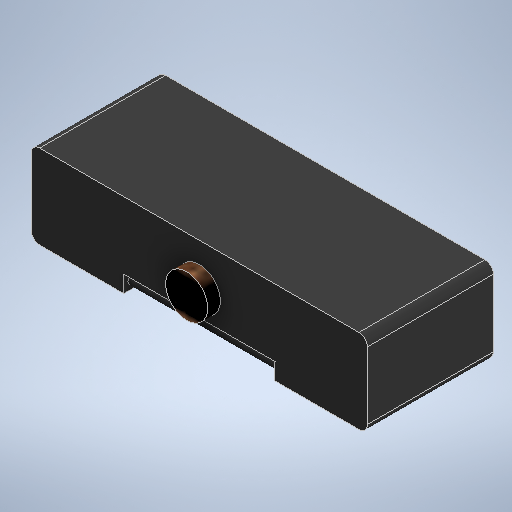
# Autodesk Inventor part: Caja
Saved by Autodesk Inventor 2025.2 (Build 292293000, 293)
## iProperties
Created: 2025-06-29
Part Number: Caja
Material: Rubber, Silicone
Document SubType Name: Sheet Metal
Designer: asus
Mass: 7.5 g
Surface Area: 23 cm^2
Volume: 6 cm^3
Density: 1.25 g/cm^3
Sheet Metal Rule: Default
Appearance: Rubber - Black
Author: asus
Autodesk Inventor part; units mm, degrees
ref_plane "YZ Plane" through (0, 0, 0) normal (1, 0, 0) x (0, 1, 0)
ref_plane "XZ Plane" through (0, 0, 0) normal (0, 1, 0) x (-1, 0, 0)
ref_plane "XY Plane" through (0, 0, 0) normal (0, 0, 1) x (1, 0, 0)
sketch "Sketch1" plane through (0, 0, 0) normal (0, 0, 1) x (1, 0, 0)
  line L0 (0, 1) -> (0, 9)
  line L1 (1, 10) -> (39, 10)
  line L2 (40, 9) -> (40, 1)
  line L3 (39, 0) -> (1, 0)
  arc A0 (1, 10) -> (0, 9) centre (1, 9) ccw
  arc A1 (40, 9) -> (39, 10) centre (39, 9) ccw
  arc A2 (39, 0) -> (40, 1) centre (39, 1) ccw
  arc A3 (0, 1) -> (1, 0) centre (1, 1) ccw
  point P0 (0, 0)
  point P1 (0, 10)
  point P2 (40, 10)
  point P3 (40, 0)
  dimension "d0" = 10
  dimension "d1" = 40
  dimension "d4" = 1
  constraints: 8 end point, 8 point on circle, 8 point on line, 8 tangent, 4 centre point, 3 equal radius, 2 perpendicular, 1 horizontal, 1 vertical
  measures "d0" distance of point (0, 0) point (0, 10)
  measures "d1" distance of point (0, 10) point (40, 10)
  measures "d4" radius of A0
extrude "Extrusion1" add sketch "Sketch1" against normal blind 15
sketch "Sketch2" plane through (1, 0, 0) normal (0, -1, 0) x (1, 0, 0)
  line L0 (0, 0) -> (38, 0) projected
  line L1 (0, 0) -> (0, -15) projected
  line L2 (38, -15) -> (0, -15) projected
  line L3 (38, 0) -> (38, -15) projected
  line L4 (0, 0) -> (38, 0) projected
  line L5 (0, 0) -> (0, -15) projected
  line L6 (38, -15) -> (0, -15) projected
  line L7 (38, 0) -> (38, -15) projected
  line L8 (0, 0) -> (38, 0) projected
  line L9 (38, -15) -> (0, -15) projected
  line L10 (0, 0) -> (0, -15) projected
  line L11 (38, 0) -> (38, -15) projected
  line L12 (16.2, -5.85) -> (16.2, -9.15)
  line L13 (16.2, -9.15) -> (21.8, -9.15)
  line L14 (21.8, -9.15) -> (21.8, -5.85)
  line L15 (21.8, -5.85) -> (16.2, -5.85)
  point P0 (-1, 0)
  point P1 (16.2, -7.5)
  dimension "d8" = 3.3
  dimension "d9" = 5.6
  dimension "d10" = 16.2
  dimension "d11" = 5.85
  constraints: 8 end point, 3 perpendicular, 1 midpoint, 1 vertical
  measures "d8" distance of L12.start L12.end
  measures "d9" distance of L12.end L13.end
  measures "d10" distance from line of point (16.2, -7.5) L1
  measures "d11" distance between parallel lines of L0 L15
extrude "Extrusion2" cut sketch "Sketch2" against normal blind 1.6 contours L15 L14 L13 L12
sketch "Sketch3" plane through (0, 0, 0) normal (0, 0, 1) x (1, 0, 0)
  line L0 (40, 1) -> (40, 9) projected
  arc A0 (40, 9) -> (39, 10) centre (39, 9) ccw projected
  line L1 (39, 10) -> (1, 10) projected
  arc A1 (1, 10) -> (0, 9) centre (1, 9) ccw projected
  line L2 (0, 9) -> (0, 1) projected
  arc A2 (0, 1) -> (1, 0) centre (1, 1) ccw projected
  line L3 (1, 0) -> (39, 0) projected
  arc A3 (39, 0) -> (40, 1) centre (39, 1) ccw projected
  circle A4 centre (20, 5) radius 2.5
  point P0 (0, 0)
  dimension "d14" = 5
  constraints: 1 centre point
  measures "d14" diameter of A4
extrude "Extrusion3" add sketch "Sketch3" along normal blind 1.5 contours A4
sketch "Sketch4" plane through (0, 0, 0) normal (0, 0, 1) x (1, 0, 0)
  line L0 (17.2, 0) -> (22.8, 0) projected
  line L1 (20, 0) -> (11, 0)
  line L2 (1, 0) -> (39, 0) projected
  line L3 (11, 0) -> (11, 2)
  line L4 (11, 2) -> (29, 2)
  line L5 (29, 2) -> (29, 0)
  line L6 (29, 0) -> (20, 0)
  point P0 (0, 0)
  point P1 (29, 0)
  dimension "d17" = 9
  dimension "d18" = 2
  dimension "d19" = 18
  constraints: 10 end point, 3 perpendicular, 2 point on line, 1 collinear, 1 midpoint
  measures "d17" distance of L1.start L1.end
  measures "d18" distance of L1.end L3.end
  measures "d19" distance of L3.end L4.end
extrude "Extrusion4" cut sketch "Sketch4" against normal blind 2
sketch "Sketch5" plane through (0, 0, -15) normal (0, 0, -1) x (-1, 0, 0)
  line L0 (-11, 2) -> (-29, 2) projected
  line L1 (-11, 0) -> (-11, 2) projected
  line L2 (-39, 0) -> (-1, 0) projected
  line L3 (-29, 2) -> (-29, 0) projected
  point P0 (0, 0)
extrude "Extrusion5" cut sketch "Sketch5" against normal blind 2
sketch "Sketch6" plane through (11, 0, 0) normal (1, 0, 0) x (0, 0, -1)
  circle A0 centre (1.0103, 0.9523) radius 0.5
  point P0 (0, 0)
  dimension "d24" = 1
  constraints: 1 centre point
  measures "d24" diameter of A0
extrude "Extrusion6" add sketch "Sketch6" along normal blind 18
sketch "Sketch7" plane through (11, 0, -15) normal (1, 0, 0) x (0, 0, -1)
  circle A0 centre (-0.8887, 1) radius 0.5
  point P0 (-15, 0)
  dimension "d27" = 1
  constraints: 1 centre point
  measures "d27" diameter of A0
extrude "Extrusion7" add sketch "Sketch7" along normal blind 18
equation "\"BendRadius\" = Thickness"
equation "\"BendReliefWidth\" = Thickness"
equation "\"BendReliefDepth\" = 0.5 * Thickness"
equation "\"CornerReliefSize\" = 4 * Thickness"
equation "\"MinimumRemnant\" = 2 * Thickness"
equation "\"TransitionRadius\" = BendRadius"
equation "\"JacobiRadiusSize\" = BendRadius"
equation "\"GapSize\" = Thickness"
equation "\"Thickness\" = 3.048"
body "Solid1"
